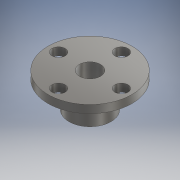
# Autodesk Inventor part: 8mm Mounting Hub
Saved by Autodesk Inventor 2017 (Build 210142000, 142)
## iProperties
Created: 2019-09-19
Part Number: 8mm Mounting Hub
Material: Steel, Mild
Document SubType Name: Modeling
Designer: Dell
Density: 7.85 g/cm^3
Appearance: Semi-Polished
Author: Dell
Autodesk Inventor part; units mm, degrees
ref_plane "YZ Plane" through (0, 0, 0) normal (1, 0, 0) x (0, 1, 0)
ref_plane "XZ Plane" through (0, 0, 0) normal (0, 1, 0) x (-1, 0, 0)
ref_plane "XY Plane" through (0, 0, 0) normal (0, 0, 1) x (1, 0, 0)
sketch "Sketch1" plane through (0, 0, 0) normal (0, 0, 1) x (1, 0, 0)
  circle A0 centre (0, 0) radius 4
  circle A1 centre (0, 0) radius 8
  dimension "d0" = 8
  dimension "d1" = 16
  constraints: 2 centre point, 2 coincident
  measures "d0" diameter of A0
  measures "d1" diameter of A1
extrude "Extrusion1" add sketch "Sketch1" along normal blind 13
sketch "Sketch2" plane through (0, 0, 13) normal (0, 0, 1) x (1, 0, 0)
  circle A0 centre (0, 0) radius 16
  circle A1 centre (0, 0) radius 8 projected
  dimension "d4" = 32
  constraints: 1 centre point, 1 coincident
  measures "d4" diameter of A0
extrude "Extrusion2" add sketch "Sketch2" against normal blind 3
sketch "Sketch3" plane through (0, 0, 13) normal (0, 0, 1) x (1, 0, 0)
  circle A0 centre (12, 0) radius 2.5
  circle A1 centre (0, 12) radius 2.5
  circle A2 centre (-12, 0) radius 2.5
  circle A3 centre (0, -12) radius 2.5
  point P0 (0, 0)
  dimension "d7" = 5
  dimension "d8" = 12
  dimension "d11" = 360
  constraints: 4 centre point, 1 horizontal alignment, 9 other
  measures "d7" diameter of A0
  measures "d8" distance of point (0, 0) A0.centre
extrude "Extrusion3" cut sketch "Sketch3" against normal through all
body "Solid1"
